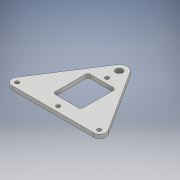
# Autodesk Inventor part: Corpo_Suporte_4_Cabos_Modelo1
Saved by Autodesk Inventor 2018 (Build 220112000, 112)
## iProperties
Created: 2021-08-02
Part Number: Corpo_Suporte_4_Cabos_Modelo1
Material: Generic
Document SubType Name: Modeling
Designer: L08619
Density: 1 g/cm^3
Appearance: Default
Author: L08619
Autodesk Inventor part; units mm, degrees
ref_plane "YZ Plane" through (0, 0, 0) normal (1, 0, 0) x (0, 1, 0)
ref_plane "XZ Plane" through (0, 0, 0) normal (0, 1, 0) x (-1, 0, 0)
ref_plane "XY Plane" through (0, 0, 0) normal (0, 0, 1) x (1, 0, 0)
sketch "Sketch1" plane through (0, 0, 0) normal (0, 0, 1) x (1, 0, 0)
  circle A0 centre (0, 0) radius 20
  circle A1 centre (0, -350) radius 11
  circle A2 centre (-235, -350) radius 11
  circle A3 centre (235, -350) radius 11
  line L0 (-233.6625, -380) -> (233.6625, -380)
  arc A4 (233.6625, -380) -> (260.9808, -323.1206) centre (233.6625, -345) ccw
  circle A5 centre (0.0008, -70) radius 11
  line L1 (70, -100) -> (-70, -100)
  line L2 (-80, -110) -> (-80, -290)
  line L3 (-70, -300) -> (70, -300)
  line L4 (80, -290) -> (80, -110)
  line L5 (80, -100) -> (-80, -300) construction
  line L6 (-80, -100) -> (80, -300) construction
  line L7 (0, 64.9697) -> (0, -492.5476)
  arc A6 (-260.9808, -323.1206) -> (-233.6625, -380) centre (-233.6625, -345) ccw
  line L8 (-80, -110) -> (-70, -100)
  line L9 (80, -110) -> (70, -100)
  line L10 (70, -300) -> (80, -290)
  line L11 (-70, -300) -> (-80, -290)
  line L12 (-260.9808, -323.1206) -> (-36.0446, 26.9405)
  arc A7 (36.0446, 26.9405) -> (-36.0446, 26.9405) centre (0, 0) ccw
  line L13 (260.9808, -323.1206) -> (36.0446, 26.9405)
  point P0 (0, -200)
  point P1 (0, -200)
  dimension "d0" = 40
  dimension "d2" = 22
  dimension "d3" = 22
  dimension "d4" = 22
  dimension "d7" = 235
  dimension "d8" = 235
  dimension "d9" = 35
  dimension "d11" = 30
  dimension "d33" = 22
  dimension "d34" = 350
  dimension "d35" = 160
  dimension "d36" = 200
  dimension "d37" = 70
  dimension "d38" = 30
  dimension "d39" = 10
  dimension "d40" = 10
  dimension "d41" = 10
  dimension "d42" = 10
  dimension "d43" = 10
  dimension "d44" = 10
  dimension "d45" = 10
  dimension "d46" = 10
  dimension "d47" = 45
  constraints: 28 end point, 8 centre point, 8 point on line, 6 point on circle, 3 midpoint, 2 coincident, 2 horizontal alignment, 2 parallel, 2 symmetric about line, 2 vertical alignment, 1 horizontal, 1 perpendicular, 1 tangent, 1 vertical, 1 other
  measures "d0" diameter of A0
  measures "d2" diameter of A1
  measures "d3" diameter of A2
  measures "d4" diameter of A3
  measures "d7" distance of A1.centre A2.centre
  measures "d8" distance of A3.centre A1.centre
  measures "d9" radius of A4
  measures "d11" distance from line of L0 A1.centre
  measures "d33" diameter of A5
  measures "d34" distance of A1.centre A0.centre
  measures "d35" distance of L5.start L6.start
  measures "d36" distance of L6.start L5.end
  measures "d37" distance of A5.centre A0.centre
  measures "d38" distance from line of L1 A5.centre
  measures "d39" distance of L2.start L6.start
  measures "d40" distance of L1.end L6.start
  measures "d41" distance of L4.end L5.start
  measures "d42" distance of L1.start L5.start
  measures "d43" distance of L3.end L6.end
  measures "d44" distance of L4.start L6.end
  measures "d45" distance of L3.start L5.end
  measures "d46" distance of L2.end L5.end
  measures "d47" radius of A7
extrude "Extrusion2" add sketch "Sketch1" along normal mid plane 22.22 contours A0 L7 A7 L13 A4 L0 A1 L3 L10 L4 L9 L1 A5 | A0 L7 A5 L1 L8 L2 L11 L3 A1 L0 A6 L12 A7
equation "\"d8\" = d7"
equation "\"d40\" = d39"
equation "\"d42\" = d41"
equation "\"d43\" = d41"
equation "\"d44\" = d43"
equation "\"d45\" = d41"
equation "\"d46\" = d45"
body "Solid2"
